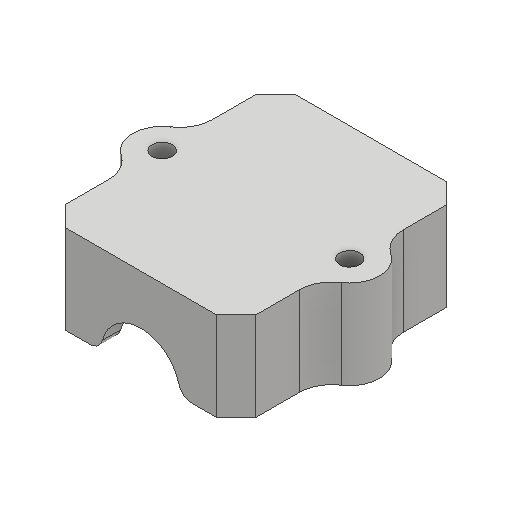
# Autodesk Inventor part: 3DP_ABS_Y_Axis_Linear_Bearing_Mount_Top
Saved by Autodesk Inventor 2026.1 (Build 301233000, 233)
## iProperties
Created: 2017-05-25
Part Number: 3DP_ABS_Y_Axis_Linear_Bearing_Mount_Top
Material: Ogólny
Document SubType Name: Modeling
Designer: Andrzej
Density: 1 g/cm^3
Appearance: Domyślna
Mass: 9.57924 g
Surface Area: 44.8006 cm^2
Volume: 9.57924 cm^3
Author: Andrzej
Autodesk Inventor part; units mm, degrees
ref_plane "YZ Plane" through (0, 0, 0) normal (1, 0, 0) x (0, 1, 0)
ref_plane "XZ Plane" through (0, 0, 0) normal (0, 1, 0) x (-1, 0, 0)
ref_plane "XY Plane" through (0, 0, 0) normal (0, 0, 1) x (1, 0, 0)
sketch "Szkic1" plane through (0, 0, 0) normal (0, 0, 1) x (1, 0, 0)
  line L0 (-13.3884, 18.62) -> (15.6116, 18.62)
  line L1 (15.6116, 18.62) -> (15.6116, -16.38)
  line L2 (15.6116, -16.38) -> (-13.3884, -16.38)
  line L3 (-13.3884, -16.38) -> (-13.3884, 18.62)
  arc A0 (-13.3884, 5.6124) -> (-13.3884, -3.3724) centre (-13.1267, 1.12) ccw
  arc A1 (15.6116, -3.3737) -> (15.6116, 5.6137) centre (15.3733, 1.12) ccw
  point P0 (0, 0)
  dimension "d2" = 35
  dimension "d5" = 28.5
  dimension "d6" = 29
  dimension "d7" = 17.5
  dimension "d8" = 17.5
  dimension "d9" = 9
  dimension "d10" = 9
  constraints: 8 end point, 4 point on circle, 4 point on line, 2 centre point, 2 coincident, 2 parallel, 1 horizontal, 1 perpendicular
  measures "d2" distance of L0.end L1.end
  measures "d5" distance of point (15.373, 1.12) point (-13.127, 1.12)
  measures "d6" distance between parallel lines of L1 L3
  measures "d7" distance from line of L0 point (-13.127, 1.12)
  measures "d8" distance from line of L0 point (15.373, 1.12)
  measures "d9" diameter of A0
  measures "d10" diameter of A1
extrude "Wyciągnięcie proste1" add sketch "Szkic1" along normal blind 13.5
hole "Otwór1" at (-13.1267, 1.12, 0) at (15.3733, 1.12, 0) direction (0, 0, 1) diameter 3.1 end through all
sketch "Szkic2" plane through (-13.3884, -16.38, 0) normal (0, -1, 0) x (1, 0, 0)
  line L0 (29, 0) -> (0, 0) projected
  line L1 (29, 0) -> (29, 13.5) projected
  line L2 (0, 13.5) -> (29, 13.5) projected
  line L3 (0, 0) -> (0, 13.5) projected
  circle A0 centre (14.5, 0) radius 9.575
  point P0 (13.3884, 0)
  dimension "d18" = 13.5
  dimension "d19" = 14.5
  dimension "d20" = 29
  dimension "d21" = 19.15
  constraints: 1 centre point, 1 coincident
  measures "d18" distance from line of point (14.5, 0) L2
  measures "d19" distance from line of L3 point (14.5, 0)
  measures "d20" distance of L2.start L1.end
  measures "d21" diameter of A0
extrude "Wyciągnięcie proste2" cut sketch "Szkic2" against normal through all contours A0 L0 | L0 A0
sketch "Szkic3" plane through (-13.3884, -16.38, 13.5) normal (0, -1, 0) x (1, 0, 0)
  arc A0 (24.075, -13.5) -> (4.925, -13.5) centre (14.5, -13.5) ccw projected
  line L0 (29, -13.5) -> (24.075, -13.5) projected
  line L1 (29, -13.5) -> (29, 0) projected
  line L2 (0, 0) -> (29, 0) projected
  line L3 (0, -13.5) -> (0, 0) projected
  line L4 (4.925, -13.5) -> (0, -13.5) projected
  arc A1 (20.5, -13.5) -> (8.5, -13.5) centre (14.5, -13.5) ccw
  line L5 (0, -13.5) -> (4.925, -13.5) projected
  arc A2 (24.075, -13.5) -> (4.925, -13.5) centre (14.5, -13.5) ccw projected
  line L6 (4.925, -13.5) -> (24.075, -13.5)
  point P0 (13.3884, -13.5)
  dimension "d24" = 12
  constraints: 2 end point, 2 point on circle, 2 point on line, 1 centre point, 1 coincident, 1 horizontal
  measures "d24" diameter of A1
extrude "Wyciągnięcie proste3" add sketch "Szkic3" against normal blind 2.75 contours L6 A1 A0
sketch "Szkic4" plane through (-13.3884, 18.62, 13.5) normal (0, 1, 0) x (1, 0, 0)
  line L0 (8.5, 13.5) -> (4.925, 13.5) projected
  arc A0 (4.925, 13.5) -> (24.075, 13.5) centre (14.5, 13.5) ccw projected
  line L1 (24.075, 13.5) -> (20.5, 13.5) projected
  arc A1 (8.5, 13.5) -> (20.5, 13.5) centre (14.5, 13.5) ccw projected
  arc A2 (4.925, 13.5) -> (24.075, 13.5) centre (14.5, 13.5) ccw projected
  line L2 (0, 13.5) -> (4.925, 13.5) projected
  line L3 (0, 13.5) -> (0, 0) projected
  line L4 (29, 0) -> (0, 0) projected
  line L5 (29, 13.5) -> (29, 0) projected
  line L6 (24.075, 13.5) -> (29, 13.5) projected
  point P0 (13.3884, 13.5)
extrude "Wyciągnięcie proste4" add sketch "Szkic4" against normal blind 2.75 contours A1 L1 A0 L0
fillet "Zaokrąglenie1" radius 5 4 edges at (15.6116, 5.6137, 6.75) (15.6116, -3.3737, 6.75) (-13.3884, -3.3724, 6.75) (-13.3884, 5.6124, 6.75)
fillet "Zaokrąglenie2" radius 2 4 edges at (7.1116, -15.005, 0) (-4.8884, -15.005, 0) (7.1116, 17.245, 0) (-4.8884, 17.245, 0)
chamfer "Faza1" distance 3 angle 45 4 edges at (-13.3884, 18.62, 6.75) (15.6116, 18.62, 6.75) (-13.3884, -16.38, 6.75) (15.6116, -16.38, 6.75)
equation "\"d7\" = 0.5 * d2"
equation "\"d8\" = d7"
equation "\"d19\" = 0.5 * d20"
